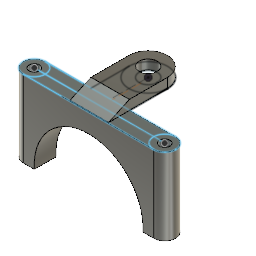
Shift P2 mount v3 (Autodesk Fusion 360 design; units mm, degrees)
Autodesk Fusion 360 part; units mm, degrees
sketch "Sketch1" plane through (0, 0, 0) normal (0, 0, 1) x (1, 0, 0)
  circle A0 centre (0, 0) radius 4.65
  circle A1 centre (0, 0) radius 10
  line L0 (-33.85, -25.2927) -> (33.85, -25.2927)
  circle A2 centre (33.85, -25.2927) radius 5.7
  circle A3 centre (-33.85, -25.2927) radius 5.7
  line L1 (-33.85, -30.9927) -> (33.85, -30.9927)
  line L2 (-33.85, -19.5927) -> (33.85, -19.5927)
  line L3 (10, -19.5927) -> (10, 0)
  line L4 (-10, -19.5927) -> (-10, 0)
  line L5 (0.7275, -4.5927) -> (0.7275, -19.5927) construction
  line L6 (0, 0) -> (0, -19.5927) construction
  dimension "d2" = 9.3
  dimension "d3" = 20
  dimension "d9" = 67.7
  dimension "d13" = 11.4
  dimension "d14" = 11.4
  dimension "d37" = 15
  constraint coincident A0.centre A1.centre
  constraint horizontal L0
  constraint coincident L0.end A2.centre
  constraint coincident L0.start A3.centre
  constraint horizontal L1
  constraint horizontal L2
  constraint coincident A3 L2.start
  constraint coincident A3 L1.start
  constraint coincident A2 L2.end
  constraint coincident A2 L1.end
  constraint coincident L2 L3.start
  constraint perpendicular L2 L3
  constraint coincident L2 L4.start
  constraint perpendicular L2 L4
  constraint tangent A1 L3
  constraint tangent A1 L4
  constraint coincident A1 L4.end
  constraint coincident A1 L3.end
  constraint coincident A0 L5.start
  constraint coincident L2 L5.end
  constraint perpendicular L2 L5
  constraint tangent A3 L2
  constraint tangent A2 L1
  constraint coincident L2 L6.end
  constraint perpendicular L2 L6
  constraint midpoint L2 L6.end
  measures "d2" diameter of A0
  measures "d3" diameter of A1
  measures "d9" distance of L0.start L0.end
  measures "d13" diameter of A2
  measures "d14" diameter of A3
  measures "d37" distance of L5.start L5.end
extrude "Extrude1" add sketch "Sketch1" along normal blind 5 contours A1 makes body 1
extrude "Extrude2" add sketch "Sketch1" along normal blind 5 contours A1 L2 L3 L4 bodies 1
extrude "Extrude3" add sketch "Sketch1" against normal blind 40 separate body contours L0 A2 A3 L2 | A2 | A3 | L0 A2 A3 L1 makes body 2
extrude "Extrude4" add 1 faces at (-3.3333, -19.5927, 1.6667) along direction (0, -1, 0) blind 0.2 on bodies 1 bodies 1 2
chamfer "Chamfer1" distance 5 distance2 10.8 1 edges at (0, -19.7927, 0) measured on face at (-3.3333, -19.7927, 1.6667) on bodies 1
hole "Hole1" at (-33.85, -25.2927, 0) at (33.85, -25.2927, 0) direction (0, 0, -1) diameter 5.4 depth 38 tip angle 180 bodies 1
hole "Hole2" at (33.85, -25.2927, -38) direction (0, 0, -1) diameter 2.65 depth 2 tip angle 180 countersink diameter 5 countersink angle 90 bodies 1
hole "Hole3" at (-33.85, -25.2927, -38) direction (0, 0, -1) diameter 2.65 depth 2 tip angle 180 countersink diameter 5 countersink angle 90 bodies 1
sketch "Sketch2" plane through (0, -30.9927, 0) normal (0, -1, 0) x (1, 0, 0)
  line L0 (33.85, 0) -> (-33.85, 0)
  line L1 (-33.85, 0) -> (-33.85, -40)
  line L2 (-33.85, -40) -> (33.85, -40)
  line L3 (33.85, -40) -> (33.85, 0)
  line L4 (-33.85, -40) -> (-28.15, -40) construction
  line L5 (33.85, -40) -> (28.15, -40) construction
  arc A0 (28.15, -40) -> (-28.15, -40) centre (0, -38.1329) ccw
  dimension "d39" = 5.7
  dimension "d40" = 5.7
  constraint coincident L1.end L2.start
  constraint perpendicular L1 L4
  constraint coincident L2.end L3.start
  constraint perpendicular L3 L5
  measures "d39" distance of L1.end L4.end
  measures "d40" distance of L2.end L5.end
extrude "Extrude5" cut sketch "Sketch2" against normal up to surface (11.4 mm away) contours L2 A0 bodies 1
equation "stemdia = 9.2 mm"
equation "d2 = stemdia + 0.1 mm"
equation "screwwidth = 67.7 mm"
equation "screwheight = 5.6 mm"
equation "d9 = screwwidth"
equation "shiftscrewdia = 2.55 mm"
equation "shiftiscrewdepth = 2 mm"
equation "d13 = standoffwidth"
equation "d14 = standoffwidth"
equation "standoff = 40 mm"
equation "d18 = -standoff"
equation "d23 = standoff - 2 mm"
equation "d36 = ( 5.5 * 2 ) * 1 mm - 0.2 mm"
equation "standoffwidth = 11.4 mm"
equation "d39 = standoffwidth / 2"
equation "d40 = standoffwidth / 2"
named bodies: "shift p2 standoff"
